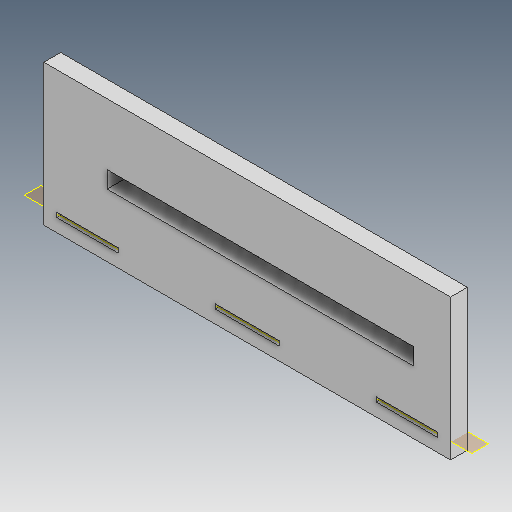
# Autodesk Inventor part: lr_bottom
Saved by Autodesk Inventor 2020 (Build 240168000, 168)
## iProperties
Created: 2021-05-08
Part Number: lr_bottom
Material: Generic
Document SubType Name: Modeling
Designer: Hsu Daniel
Density: 1 g/cm^3
Appearance: Default
Author: Hsu Daniel
Autodesk Inventor part; units mm, degrees
ref_plane "YZ Plane" through (0, 0, 0) normal (1, 0, 0) x (0, 1, 0)
sketch "Sketch1" plane through (0, 0, 0) normal (0, 0, 1) x (1, 0, 0)
  line L0 (0, 0) -> (132.6, 0)
  line L1 (132.6, 0) -> (132.6, 46)
  line L2 (132.6, 46) -> (0, 46)
  line L3 (0, 46) -> (0, 0)
  line L4 (66.3, 46) -> (66.3, 0) construction
  line L5 (55.85, 4.25) -> (76.75, 4.25)
  line L6 (76.75, 4.25) -> (76.75, 5.75)
  line L7 (76.75, 5.75) -> (55.85, 5.75)
  line L8 (55.85, 5.75) -> (55.85, 4.25)
  line L9 (55.85, 4.25) -> (76.75, 5.75) construction
  line L10 (76.75, 4.25) -> (55.85, 5.75) construction
  line L11 (4.2, 5.75) -> (24.2, 5.75)
  line L12 (24.2, 5.75) -> (24.2, 4.25)
  line L13 (24.2, 4.25) -> (4.2, 4.25)
  line L14 (4.2, 4.25) -> (4.2, 5.75)
  line L15 (4.2, 5.75) -> (24.2, 4.25) construction
  line L16 (24.2, 5.75) -> (4.2, 4.25) construction
  line L17 (108.4, 4.25) -> (128.4, 4.25)
  line L18 (128.4, 4.25) -> (128.4, 5.75)
  line L19 (128.4, 5.75) -> (108.4, 5.75)
  line L20 (108.4, 5.75) -> (108.4, 4.25)
  line L21 (108.4, 4.25) -> (128.4, 5.75) construction
  line L22 (128.4, 4.25) -> (108.4, 5.75) construction
  line L23 (14.2, 5) -> (118.4, 5) construction
  point P0 (66.3, 5)
  point P1 (66.3, 5)
  dimension "d0" = 132.6
  dimension "d1" = 46
  dimension "d2" = 1.5
  dimension "d3" = 20.9
  dimension "d4" = 1.5
  dimension "d5" = 20
  dimension "d7" = 20
  dimension "d8" = 1.5
  dimension "d17" = 5
  dimension "d18" = 52.1
  constraints: 48 end point, 9 midpoint, 8 parallel, 5 horizontal, 4 perpendicular, 1 point on line
  measures "d0" distance of L1.end L2.end
  measures "d1" distance of L0.end L1.end
  measures "d2" distance of L6.end L5.end
  measures "d3" distance of L6.end L7.end
  measures "d4" distance of L11.end L12.end
  measures "d5" distance of L11.start L11.end
  measures "d7" distance of L19.end L18.end
  measures "d8" distance of L17.end L18.end
  measures "d17" distance between parallel lines of L0 L23
  measures "d18" distance of point (66.3, 5) L23.start
extrude "Extrusion1" add sketch "Sketch1" along normal blind 5.5
ref_plane "Work Plane1" through (0, 23, 0) normal (0, 1, 0) x (1, 0, 0)
ref_plane "Work Plane2" through (66.3, 0, 0) normal (1, 0, 0) x (0, 0, -1)
ref_plane "Work Plane3" through (4.2, 5, 0) normal (0, 1, 0) x (1, 0, 0)
sketch "Sketch3" plane through (0, 0, 5.5) normal (0, 0, 1) x (1, 0, 0)
  line L0 (20.6246, 26) -> (120.6246, 26)
  line L1 (120.6246, 26) -> (120.6246, 20.5)
  line L2 (120.6246, 20.5) -> (20.6246, 20.5)
  line L3 (20.6246, 20.5) -> (20.6246, 26)
  line L4 (132.6, 46) -> (0, 46) projected
  point P0 (0, 0)
  dimension "d19" = 100
  dimension "d20" = 5.5
  dimension "d21" = 20
  constraints: 8 end point, 2 parallel, 1 horizontal, 1 perpendicular
  measures "d19" distance of L1.end L2.end
  measures "d20" distance of L0.end L1.end
  measures "d21" distance between parallel lines of L4 L0
extrude "Extrusion2" cut sketch "Sketch3" against normal blind 5.5
equation "\"d3\" = lrmid + toler"
equation "\"d4\" = d2"
equation "\"d5\" = lrlr + toler"
equation "\"d7\" = d5"
equation "\"d8\" = d2"
equation "\"d18\" = lrbetween"
equation "\"thick\" = 0.5"
equation "\"lrlr\" = 19"
equation "\"lrmid\" = 19.9"
equation "\"lrdepth\" = 3.3"
equation "\"mlr\" = 16.6"
equation "\"mmid\" = 24.7"
equation "\"mdepth\" = 4.5"
equation "\"lrltotal\" = 126.6"
equation "\"mltotal\" = 126.6"
equation "\"lrbetween\" = 52.1"
equation "\"mbetween\" = 49.5"
equation "\"toler\" = 1"
equation "\"stuckw\" = 6"
equation "\"tight\" = 0.08"
equation "\"sidewallL\" = 132.6"
equation "\"heaterH\" = 117.3"
equation "\"stickL\" = 3.5"
equation "\"wireH\" = 25"
body "Solid1"
